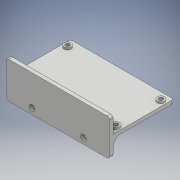
# Autodesk Inventor part: Eletronica - suporteLed
Saved by Autodesk Inventor 2017 (Build 210142000, 142)
## iProperties
Created: 2020-10-10
Part Number: Eletronica - suporteLed
Material: Generic
Document SubType Name: Modeling
Designer: ale
Density: 1 g/cm^3
Appearance: Default
Author: ale
Autodesk Inventor part; units mm, degrees
ref_plane "YZ Plane" through (0, 0, 0) normal (1, 0, 0) x (0, 1, 0)
ref_plane "XZ Plane" through (0, 0, 0) normal (0, 1, 0) x (-1, 0, 0)
ref_plane "XY Plane" through (0, 0, 0) normal (0, 0, 1) x (1, 0, 0)
sketch "Sketch1" plane through (0, 0, 0) normal (0, 0, 1) x (1, 0, 0)
  line L0 (-42.5, 25) -> (42.5, 25)
  line L1 (42.5, 25) -> (42.5, -25)
  line L2 (42.5, -25) -> (-42.5, -25)
  line L3 (-42.5, -25) -> (-42.5, 25)
  line L4 (-42.5, 25) -> (42.5, -25) construction
  line L5 (42.5, 25) -> (-42.5, -25) construction
  point P0 (0, 0)
  dimension "d0" = 85
  dimension "d1" = 50
  constraints: 12 end point, 2 midpoint, 2 parallel, 1 horizontal, 1 perpendicular
  measures "d0" distance of L1.end L2.end
  measures "d1" distance of L0.end L1.end
extrude "Extrusion1" add sketch "Sketch1" along normal blind 3
sketch "Sketch2" plane through (0, 0, 3) normal (0, 0, 1) x (1, 0, 0)
  line L0 (-38.5, 18.5) -> (38.5, 18.5)
  line L1 (38.5, 18.5) -> (38.5, -18.5)
  line L2 (38.5, -18.5) -> (-38.5, -18.5)
  line L3 (-38.5, -18.5) -> (-38.5, 18.5)
  line L4 (-38.5, 18.5) -> (38.5, -18.5) construction
  line L5 (38.5, 18.5) -> (-38.5, -18.5) construction
  circle A0 centre (-38.5, 18.5) radius 3
  circle A1 centre (38.5, 18.5) radius 3
  circle A2 centre (38.5, -18.5) radius 3
  circle A3 centre (-38.5, -18.5) radius 3
  point P0 (0, 0)
  dimension "d4" = 77
  dimension "d5" = 37
  dimension "d6" = 6
  dimension "d7" = 6
  dimension "d8" = 6
  dimension "d9" = 6
  constraints: 12 end point, 4 centre point, 4 coincident, 2 midpoint, 2 parallel, 1 horizontal, 1 perpendicular
  measures "d4" distance of L1.end L2.end
  measures "d5" distance of L0.end L1.end
  measures "d6" diameter of A0
  measures "d7" diameter of A1
  measures "d8" diameter of A2
  measures "d9" diameter of A3
extrude "Extrusion2" add sketch "Sketch2" along normal blind 1.5 contours L3 A0 L0 | L0 A0 L3 | A1 L1 L0 | L0 L1 A1 | A3 L2 L3 | L3 L2 A3 | A2 L2 L1 | L1 L2 A2
sketch "Sketch3" plane through (-38.5, 18.5, 4.5) normal (0, 0, 1) x (1, 0, 0)
  circle A0 centre (0, 0) radius 3 projected
  circle A1 centre (77, 0) radius 3 projected
  circle A2 centre (77, -37) radius 3 projected
  circle A3 centre (0, -37) radius 3 projected
  point P0 (38.5, -18.5)
  constraints: 4 coincident
hole "Hole1" at (-38.5, 18.5, 4.5) at (38.5, 18.5, 4.5) at (38.5, -18.5, 4.5) at (-38.5, -18.5, 4.5) direction (0, 0, -1) diameter 3.5 end through all
sketch "Sketch4" plane through (-42.5, -25, 0) normal (0, -1, 0) x (1, 0, 0)
  line L0 (0, 0) -> (0, 3) projected
  line L1 (0, 1.5) -> (85, 1.5)
  line L2 (85, 0) -> (0, 0) projected
  line L3 (0, 16.5) -> (85, 16.5)
  line L4 (85, 16.5) -> (85, -13.5)
  line L5 (85, -13.5) -> (0, -13.5)
  line L6 (0, -13.5) -> (0, 16.5)
  line L7 (0, 16.5) -> (85, -13.5) construction
  line L8 (85, 16.5) -> (0, -13.5) construction
  point P0 (42.5, 0)
  point P1 (42.5, 1.5)
  dimension "d19" = 85
  dimension "d20" = 30
  constraints: 14 end point, 4 midpoint, 3 parallel, 1 horizontal, 1 perpendicular
  measures "d19" distance of L4.end L5.end
  measures "d20" distance of L3.end L4.end
extrude "Extrusion3" add sketch "Sketch4" along normal blind 3
chamfer "Chamfer1" distance 4 angle 45 1 edges at (0, -25, 0)
sketch "Sketch5" plane through (-42.5, -25, 0) normal (0, 1, 0) x (1, 0, 0)
  line L0 (85, 13.5) -> (0, 13.5) projected
  line L1 (85, 4) -> (85, 13.5) projected
  point P0 (42.5, 0)
  point P1 (63.75, 8.75)
  point P2 (21.25, 8.75)
  dimension "d26" = 4.75
  dimension "d27" = 4.75
  dimension "d28" = 21.25
  dimension "d29" = 63.75
  measures "d26" distance from line of L0 point (63.75, 8.75)
  measures "d27" distance from line of L0 point (21.25, 8.75)
  measures "d28" distance from line of L1 point (63.75, 8.75)
  measures "d29" distance from line of point (21.25, 8.75) L1
hole "Hole2" at (21.25, -25, -8.75) at (-21.25, -25, -8.75) direction (0, -1, 0) diameter 5 end through all
fillet "Fillet1" radius 2 6 edges at (42.5, 25, 1.5) (-42.5, 25, 1.5) (-42.5, -26.5, -13.5) (42.5, -26.5, -13.5) (42.5, -26.5, 16.5) (-42.5, -26.5, 16.5)
body "Solid1"
